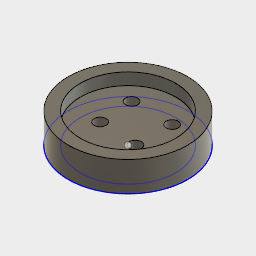
666 (Autodesk Fusion 360 design; units mm, degrees)
Autodesk Fusion 360 part; units mm, degrees
sketch "草图1" plane through (0, 0, 0) normal (0, 1, 0) x (1, 0, 0)
  circle A0 centre (50, -50) radius 10
  circle A1 centre (50, -50) radius 8
  dimension "d1" = 2
extrude "拉伸1" add sketch "草图1" along normal blind 3 contours A1 makes body 1
extrude "拉伸2" add sketch "草图1" along normal blind 5 separate body makes body 2
sketch "草图2" plane through (0, 0, 0) normal (0, 1, 0) x (1, 0, 0)
cylinder "圆柱体基本要素1" add diameter 2 height 20 placed x (1, 0, 0) y (0, 0, -1) z (0, 1, 0) at (25, 0, 50) separate body makes body 3
pattern_circular "C-阵列1" count 4 over 360 about axis through (25, 0, 50) along (0, 1, 0) of bodies 3 makes body 4 at (25.0996, 13.3333, 49.005) makes body 5 at (25.9397, 6.6667, 49.658) makes body 6 at (24.9004, 13.3333, 50.995)
cylinder "圆柱体基本要素2" add diameter 2 height 20 placed x (1, 0, 0) y (0, 0, -1) z (0, 1, 0) at (30, 0, 35) separate body makes body 7
cylinder "圆柱体基本要素3" add diameter 2 height 20 placed x (1, 0, 0) y (0, 0, -1) z (0, 1, 0) at (30, 0, 60) separate body makes body 8
cylinder "圆柱体基本要素4" add diameter 2 height 20 placed x (1, 0, 0) y (0, 0, -1) z (0, 1, 0) at (30, 0, 50) separate body makes body 9
move_face "MoveFace1" to x (1, 0, 0) y (0, 1, 0) z (0, 0, 1) at (17.5872, -7.3189, 11.3338) 1 faces at (29.0603, 6.6667, 35.342) on bodies 7
move_face "MoveFace2" by (0.9831, 0.9831, 0) 1 faces at (47.8809, 20, 46.1145) on bodies 7
move_body "移动1" bodies 7 to x (1, 0, 0) y (0, 1, 0) z (0, 0, 1) at (-0.6554, -4.0418, 0)
move_body "移动2" bodies 9 to x (1, 0, 0) y (0, 1, 0) z (0, 0, 1) at (23.7046, -2.6217, -3.7141)
move_body "移动3" bodies 4 6 5 3 to x (1, 0, 0) y (0, 1, 0) z (0, 0, 1) at (22.2845, -3.0587, 1.9663)
move_body "移动4" bodies 8 to x (1, 0, 0) y (0, 1, 0) z (0, 0, 1) at (23.5953, -3.8233, -7.6466)
combine "合并1" operation cut target body 1 tool bodies 7 9 8 6
combine "合并2" operation cut target body 1 tool bodies 3
combine "合并3" operation cut target body 1 tool bodies 4
combine "合并4" operation cut target body 1 tool bodies 5
